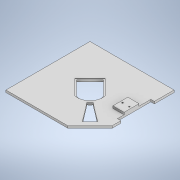
# Autodesk Inventor part: Drop_Plate
Saved by Autodesk Inventor 2022 (Build 260153000, 153)
## iProperties
Created: 2023-02-27
Part Number: Drop_Plate
Material: Generic
Document SubType Name: Modeling
Designer: zarek
Density: 1 g/cm^3
Appearance: Default
Author: zarek
Autodesk Inventor part; units mm, degrees
ref_plane "YZ Plane" through (0, 0, 0) normal (1, 0, 0) x (0, 1, 0)
ref_plane "XZ Plane" through (0, 0, 0) normal (0, 1, 0) x (-1, 0, 0)
ref_plane "XY Plane" through (0, 0, 0) normal (0, 0, 1) x (1, 0, 0)
sketch "Sketch1" plane through (0, 0, 0) normal (0, 1, 0) x (-1, 0, 0)
  line L0 (101.6, -101.6) -> (-101.6, -101.6)
  line L1 (-101.6, -101.6) -> (-101.6, 101.6)
  line L2 (-101.6, 101.6) -> (101.6, 101.6)
  line L3 (101.6, 101.6) -> (101.6, -101.6)
  line L4 (96.6, -96.6) -> (-96.6, -96.6)
  line L5 (-96.6, -96.6) -> (-96.6, 96.6)
  line L6 (-96.6, 96.6) -> (96.6, 96.6)
  line L7 (96.6, 96.6) -> (96.6, -96.6)
  line L8 (101.6, 101.6) -> (-40.4, 101.6)
  circle A0 centre (0, 0) radius 88.9
  line L9 (-40.4, 101.6) -> (-101.6, 40.4)
  line L10 (-45.4, 101.6) -> (-101.6, 45.4)
  line L11 (96.6, 96.6) -> (96.6, 101.6)
  line L12 (-45.4, 101.6) -> (-35.4, 101.6)
  line L13 (-35.4, 101.6) -> (-35.4, 96.6)
  line L14 (-35.4, 96.6) -> (-45.4, 96.6)
  line L15 (-45.4, 96.6) -> (-45.4, 101.6)
  line L16 (-101.6, 39.4) -> (-39.4, 101.6)
  line L17 (95.6, -95.6) -> (-95.6, -95.6)
  line L18 (-95.6, -95.6) -> (-95.6, 95.6)
  line L19 (-95.6, 95.6) -> (95.6, 95.6)
  line L20 (95.6, 95.6) -> (95.6, -95.6)
  point P0 (96.6, 51.2168)
  point P1 (101.6, 40.4)
  point P2 (101.6, -40.4)
  point P3 (96.6, -51.2168)
  point P4 (-96.6, 45.4)
  point P5 (-45.4, 96.6)
  point P6 (-45.4, 95.6)
  point P7 (-95.6, 45.4)
  dimension "d0" = 203.2
  dimension "d1" = 203.2
  dimension "d2" = 101.6
  dimension "d3" = 101.6
  dimension "d4" = 5
  dimension "d5" = 5
  dimension "d6" = 5
  dimension "d7" = 5
  dimension "d8" = 142
  dimension "d9" = 61.2
  dimension "d10" = 177.8
  dimension "d11" = 5
  dimension "d12" = 5
  dimension "d13" = 10
  dimension "d14" = 1
  dimension "d15" = 1
  dimension "d16" = 1
  dimension "d17" = 1
  dimension "d18" = 1
  constraints: 42 end point, 10 parallel, 8 point on line, 5 perpendicular, 4 horizontal, 1 centre point, 1 coincident
  measures "d0" distance between parallel lines of L2 L0
  measures "d1" distance between parallel lines of L1 L3
  measures "d2" distance from line of L0 point (0, 0)
  measures "d3" distance from line of L1 point (0, 0)
  measures "d4" distance between parallel lines of L4 L0
  measures "d5" distance between parallel lines of L1 L5
  measures "d6" distance between parallel lines of L2 L6
  measures "d7" distance between parallel lines of L3 L7
  measures "d8" distance of L2.end L8.end
  measures "d9" distance from line of L1 L8.end
  measures "d10" diameter of A0
  measures "d11" distance of L10.end L9.end
  measures "d12" distance of L10.start L8.end
  measures "d13" distance of L13.end L14.end
  measures "d14" distance of L9.end L16.start
  measures "d15" distance between parallel lines of L5 L18
  measures "d16" distance between parallel lines of L4 L17
  measures "d17" distance between parallel lines of L7 L20
  measures "d18" distance between parallel lines of L6 L19
extrude "Extrusion1" add sketch "Sketch1" along normal blind 5 contours L16 L19 L20 L17 L18 | A0
sketch "Sketch2" plane through (0, 5, 0) normal (0, 1, 0) x (1, 0, 0)
  circle A0 centre (0, 0) radius 34.925
  circle A1 centre (0, 0) radius 88.9
  line L0 (0, 0) -> (53.5014, -70.9987)
  line L1 (0, 0) -> (70.9987, -53.5014)
  line L2 (45.4, -95.6) -> (95.6, -45.4) projected
  line L3 (70.5, -70.5) -> (0, 0)
  point P0 (21.0184, -27.8923)
  point P1 (27.8923, -21.0184)
  dimension "d21" = 69.85
  dimension "d22" = 177.8
  dimension "d23" = 8
  dimension "d24" = 8
  constraints: 6 end point, 2 centre point, 2 coincident, 2 point on circle, 1 midpoint, 1 perpendicular
  measures "d21" diameter of A0
  measures "d22" diameter of A1
  measures "d23" angle of L1 L3
  measures "d24" angle of L0 L3
extrude "Extrusion2" cut sketch "Sketch2" against normal blind 5 contours A0 L3 A1 L0 | L1 A1 L3 A0
sketch "Sketch3" plane through (0, 5, 0) normal (0, 1, 0) x (1, 0, 0)
  circle A0 centre (0, 0) radius 2.5
  line L0 (11.3314, 2.139) -> (-2.139, -11.3314)
  line L1 (0, 0) -> (-5.6569, 5.6569)
  line L2 (-5.6569, -14.8492) -> (-26.163, 5.6569)
  line L3 (-5.6569, 26.163) -> (14.8492, 5.6569)
  circle A1 centre (-5.6569, 5.6569) radius 14
  line L4 (-26.163, 5.6569) -> (-5.6569, 26.163)
  line L5 (14.8492, 5.6569) -> (-5.6569, -14.8492)
  line L6 (-40.3051, 5.6569) -> (-5.6569, 40.3051)
  line L7 (-5.6569, 40.3051) -> (28.9914, 5.6569)
  line L8 (28.9914, 5.6569) -> (-5.6569, -28.9914)
  line L9 (-5.6569, -28.9914) -> (-40.3051, 5.6569)
  line L10 (-22.6451, 9.1747) -> (-9.1747, 22.6451)
  line L11 (-9.1747, 22.6451) -> (-12.7668, 26.2372)
  line L12 (-12.7668, 26.2372) -> (-26.2372, 12.7668)
  line L13 (-26.2372, 12.7668) -> (-22.6451, 9.1747)
  line L14 (-36.0624, 5.6569) -> (-5.6569, 36.0624)
  line L15 (-5.6569, 36.0624) -> (26.8701, 3.5355)
  line L16 (26.8701, 3.5355) -> (-3.5355, -26.8701)
  line L17 (-3.5355, -26.8701) -> (-36.0624, 5.6569)
  arc A2 (-5.6569, -28.9914) -> (28.9914, 5.6569) centre (0.4206, -0.4206) ccw
  dimension "d27" = 8
  dimension "d28" = 28
  dimension "d29" = 29
  dimension "d30" = 29
  dimension "d31" = 14.5
  dimension "d32" = 10
  dimension "d33" = 10
  dimension "d34" = 10
  dimension "d35" = 10
  dimension "d36" = 5.08
  dimension "d37" = 9.525
  dimension "d38" = 9.525
  dimension "d39" = 3
  dimension "d40" = 3
  dimension "d41" = 0
  dimension "d42" = 3
  dimension "d51" = 29.21
  constraints: 36 end point, 8 parallel, 4 perpendicular, 3 centre point, 2 coincident, 2 point on circle, 2 point on line
  measures "d27" distance of L1.start L1.end
  measures "d28" diameter of A1
  measures "d29" distance between parallel lines of L5 L4
  measures "d30" distance between parallel lines of L3 L2
  measures "d31" distance from line of A1.centre L4
  measures "d32" distance between parallel lines of L7 L3
  measures "d33" distance between parallel lines of L4 L6
  measures "d34" distance between parallel lines of L9 L2
  measures "d35" distance between parallel lines of L8 L5
  measures "d36" distance between parallel lines of L10 L12
  measures "d37" distance from line of A1.centre L11
  measures "d38" distance from line of L1.end L13
  measures "d39" distance between parallel lines of L14 L6
  measures "d40" distance between parallel lines of L9 L17
  measures "d41" distance between parallel lines of L8 L16
  measures "d42" distance between parallel lines of L7 L15
  measures "d51" radius of A2
extrude "Extrusion3" cut sketch "Sketch3" against normal blind 1 contours A0 | L0 L5 L2 L4 L3 | L4 L13 L12 L11 | A1 | L6 L7 L8 L15 L14 L17 L9 | L8 A2 | L17 L14 L15 L8
sketch "Sketch4" plane through (0, 4, 0) normal (0, 1, 0) x (1, 0, 0)
  line L0 (-36.0624, 5.6569) -> (-5.6569, 36.0624)
  line L1 (-5.6569, 36.0624) -> (26.8701, 3.5355)
  line L2 (26.8701, 3.5355) -> (-3.5355, -26.8701)
  line L3 (-3.5355, -26.8701) -> (-36.0624, 5.6569)
  line L4 (-5.6569, 40.3051) -> (28.9914, 5.6569) projected
  line L5 (-40.3051, 5.6569) -> (-5.6569, 40.3051) projected
  line L6 (-5.6569, -28.9914) -> (-40.3051, 5.6569) projected
  line L7 (28.9914, 5.6569) -> (-5.6569, -28.9914) projected
  arc A0 (-3.5355, -26.8701) -> (26.8701, 3.5355) centre (4.0877, -4.0877) ccw
  point P0 (0, 0)
  dimension "d45" = 3
  dimension "d46" = 3
  dimension "d47" = 3
  dimension "d48" = 0
  constraints: 8 end point, 2 parallel, 2 point on circle, 1 centre point, 1 perpendicular, 1 other
  measures "d45" distance between parallel lines of L4 L1
  measures "d46" distance between parallel lines of L0 L5
  measures "d47" distance between parallel lines of L6 L3
  measures "d48" distance between parallel lines of L7 L2
extrude "Extrusion4" cut sketch "Sketch4" against normal blind 5 contours L0 L1 L2 L3 | L2 A0
sketch "Sketch6" plane through (0, 5, 0) normal (0, 1, 0) x (1, 0, 0)
  line L0 (95.6, 95.6) -> (-95.6, 95.6) projected
  line L1 (95.6, 95.6) -> (87.6, 95.6)
  line L2 (87.6, 95.6) -> (87.6, -46.4)
  line L3 (87.6, -46.4) -> (95.6, -46.4)
  line L4 (95.6, -46.4) -> (95.6, 95.6)
  line L5 (95.6, -45.4) -> (95.6, 95.6) projected
  line L6 (87.6, -25.4) -> (95.6, -25.4)
  line L7 (95.6, -25.4) -> (95.6, 50.8)
  line L8 (95.6, 50.8) -> (87.6, 50.8)
  line L9 (87.6, 50.8) -> (87.6, -25.4)
  line L10 (0, 0) -> (95.6, 0)
  dimension "d58" = 8
  dimension "d59" = 142
  dimension "d62" = 50.8
  dimension "d63" = 25.4
  constraints: 18 end point, 4 parallel, 3 perpendicular, 3 point on line, 2 horizontal
  measures "d58" distance of L3.end L2.end
  measures "d59" distance between parallel lines of L3 L0
  measures "d62" distance between parallel lines of L10 L8
  measures "d63" distance between parallel lines of L10 L6
extrude "Extrusion6" cut sketch "Sketch6" against normal blind 25.4 contours L4 L10 L2 L8 | L4 L6 L2 L10
sketch "Sketch7" plane through (0, 5, 0) normal (0, 1, 0) x (1, 0, 0)
  line L0 (-95.6, 95.6) -> (-95.6, -95.6) projected
  line L1 (-95.6, -95.6) -> (45.4, -95.6) projected
  line L2 (95.6, 50.8) -> (87.6, 50.8) projected
  line L3 (87.6, 50.8) -> (62.2, 50.8)
  line L4 (87.6, -25.4) -> (87.6, 50.8)
  line L5 (87.6, -25.4) -> (87.6, 50.8) projected
  line L6 (87.6, 50.8) -> (95.6, 50.8) projected
  line L7 (87.6, 50.8) -> (62.2, 50.8)
  line L8 (62.2, 50.8) -> (62.2, -10.16)
  line L9 (62.2, -10.16) -> (87.6, -10.16)
  line L10 (87.6, -10.16) -> (87.6, 50.8)
  line L11 (62.2, 23.8506) -> (87.6, 23.8506)
  point P0 (0, 0)
  dimension "d72" = 60.96
  dimension "d90" = 34.0106
  constraints: 14 end point, 3 horizontal, 2 parallel, 2 point on line, 1 perpendicular
  measures "d72" distance of L8.end L7.end
  measures "d90" distance between parallel lines of L9 L11
extrude "Extrusion7" add sketch "Sketch7" along normal blind 5 contours L4 L9 L8 L11
sketch "Sketch8" plane through (0, 10, 0) normal (0, 1, 0) x (1, 0, 0)
  line L0 (48.8597, -4.3723) -> (48.8597, 15.6277)
  line L1 (14.8597, -4.3723) -> (14.8597, 15.6277)
  line L2 (48.8597, 15.6277) -> (14.8597, 15.6277)
  line L3 (31.8597, 15.6277) -> (31.8597, -4.3723)
  circle A0 centre (31.8597, 10.6277) radius 1
  circle A1 centre (31.8597, 0.6277) radius 1
  line L4 (62.2, -10.16) -> (87.6, -10.16) projected
  line L5 (62.2, -10.16) -> (87.6, -10.16)
  line L6 (87.6, -10.16) -> (87.6, 6.8326)
  line L7 (87.6, 50.8) -> (87.6, -25.4) projected
  line L8 (87.6, 6.8326) -> (62.2, 6.8326)
  circle A2 centre (82.6, 6.8326) radius 1.5
  circle A3 centre (67.2, 6.8326) radius 1.5
  point P0 (0, 0)
  dimension "d73" = 2
  dimension "d74" = 2
  dimension "d75" = 5
  dimension "d76" = 5
  dimension "d77" = 17
  dimension "d78" = 16.9926
  dimension "d79" = 3
  dimension "d80" = 3
  dimension "d81" = 5
  dimension "d82" = 5
  constraints: 14 end point, 5 point on line, 4 centre point, 1 collinear, 1 midpoint, 1 perpendicular, 1 vertical
  measures "d73" diameter of A0
  measures "d74" diameter of A1
  measures "d75" distance of A0.centre L3.start
  measures "d76" distance of L3.end A1.centre
  measures "d77" distance between parallel lines of L0 L3
  measures "d78" distance of L4.end L6.end
  measures "d79" diameter of A2
  measures "d80" diameter of A3
  measures "d81" distance of L6.end A2.centre
  measures "d82" distance of L8.end A3.centre
hole "Hole1" at (82.6, 10, -6.8326) at (67.2, 10, -6.8326) direction (0, -1, 0) diameter 2.85 depth 12.7 tip angle 118 countersink diameter 3.175 countersink angle 82 thread size "M3.5x0.6" class "6H" standard "ANSI Metric M Profile"
equation "\"d1\" = d0"
equation "\"d2\" = 0.5 * d0"
equation "\"d3\" = 0.5 * d0"
body "Solid1"
